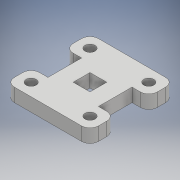
# Autodesk Inventor part: P2-8
Saved by Autodesk Inventor 2017 (Build 210142000, 142)
## iProperties
Created: 2017-02-09
Part Number: P2-8
Material: Generic
Document SubType Name: Modeling
Designer: Schaffel
Density: 1 g/cm^3
Appearance: Default
Author: Schaffel
Autodesk Inventor part; units mm, degrees
ref_plane "YZ Plane" through (0, 0, 0) normal (1, 0, 0) x (0, 1, 0)
ref_plane "XZ Plane" through (0, 0, 0) normal (0, 1, 0) x (-1, 0, 0)
ref_plane "XY Plane" through (0, 0, 0) normal (0, 0, 1) x (1, 0, 0)
sketch "Sketch1" plane through (0, 0, 0) normal (0, 0, 1) x (1, 0, 0)
  line L0 (10, 0) -> (90, 0)
  line L1 (100, 10) -> (100, 20)
  line L2 (90, 30) -> (80, 30)
  line L3 (80, 30) -> (80, 70)
  line L4 (80, 70) -> (90, 70)
  line L5 (100, 80) -> (100, 90)
  line L6 (90, 100) -> (10, 100)
  line L7 (0, 90) -> (0, 80)
  line L8 (10, 70) -> (20, 70)
  line L9 (20, 70) -> (20, 30)
  line L10 (20, 30) -> (10, 30)
  line L11 (0, 10) -> (0, 20)
  line L12 (40, 40) -> (60, 40)
  line L13 (60, 40) -> (60, 60)
  line L14 (60, 60) -> (40, 60)
  line L15 (40, 60) -> (40, 40)
  circle A0 centre (15, 15) radius 6
  circle A1 centre (85, 15) radius 6
  circle A2 centre (15, 85) radius 6
  circle A3 centre (85, 85) radius 6
  arc A4 (10, 100) -> (0, 90) centre (10, 90) ccw
  arc A5 (0, 80) -> (10, 70) centre (10, 80) ccw
  arc A6 (90, 70) -> (100, 80) centre (90, 80) ccw
  arc A7 (100, 90) -> (90, 100) centre (90, 90) ccw
  arc A8 (100, 20) -> (90, 30) centre (90, 20) ccw
  arc A9 (90, 0) -> (100, 10) centre (90, 10) ccw
  arc A10 (0, 10) -> (10, 0) centre (10, 10) ccw
  arc A11 (10, 30) -> (0, 20) centre (10, 20) ccw
  point P0 (0, 0)
  point P1 (100, 70)
  point P2 (100, 100)
  point P3 (0, 70)
  point P4 (0, 30)
  dimension "d0" = 10
  constraints: 32 end point, 17 point on line, 16 point on circle, 16 tangent, 12 centre point, 11 perpendicular, 7 equal radius, 2 horizontal
  measures "d0" radius of A4
extrude "Extrusion1" add sketch "Sketch1" along normal blind 16
body "Solid1"
